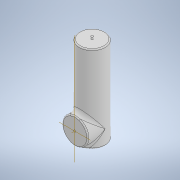
# Autodesk Inventor part: Link3
Saved by Autodesk Inventor 2021 (Build 250183000, 183)
## iProperties
Created: 2021-03-25
Part Number: Link3
Material: 일반
Document SubType Name: Modeling
Designer: jglee
Density: 1 g/cm^3
Appearance: 기본값
Author: jglee
Autodesk Inventor part; units mm, degrees
ref_plane "YZ Plane" through (0, 0, 0) normal (1, 0, 0) x (0, 1, 0)
ref_plane "XZ Plane" through (0, 0, 0) normal (0, 1, 0) x (-1, 0, 0)
ref_plane "XY Plane" through (0, 0, 0) normal (0, 0, 1) x (1, 0, 0)
sketch "스케치1" plane through (0, 0, 0) normal (0, 0, 1) x (1, 0, 0)
  circle A0 centre (0, 0) radius 60
  dimension "d0" = 120
  constraints: 1 centre point, 1 coincident
  measures "d0" diameter of A0
extrude "돌출1" add sketch "스케치1" against normal blind 80
sketch "스케치2" plane through (0, 0, 0) normal (0, 1, 0) x (-1, 0, 0)
  line L0 (-60, -80) -> (60, -80) projected
  circle A0 centre (0, -80) radius 60
  point P0 (0, 0)
  dimension "d3" = 120
  constraints: 1 centre point, 1 midpoint
  measures "d3" diameter of A0
extrude "돌출2" add sketch "스케치2" along normal blind 330 and the other way blind 70
sketch "스케치3" plane through (0, 0, 0) normal (0, 0, 1) x (1, 0, 0)
  circle A0 centre (0, 0) radius 5
  dimension "d8" = 10
  constraints: 1 centre point, 1 coincident
  measures "d8" diameter of A0
extrude "돌출3" cut sketch "스케치3" against normal blind 10
sketch "스케치4" plane through (0, 330, -80) normal (0, 1, 0) x (1, 0, 0)
  circle A0 centre (0, 0) radius 5
  point P0 (0, -80)
  dimension "d11" = 10
  constraints: 1 centre point
  measures "d11" diameter of A0
extrude "돌출4" add sketch "스케치4" along normal blind 10
fillet "모깎기1" radius 20 4 edges at (42.4264, -42.4264, -37.5736) (-42.4264, -42.4264, -37.5736) (-42.4264, 42.4264, -37.5736) (42.4264, 42.4264, -37.5736)
fillet "모깎기2" radius 5 7 edges at (60, 0, 0) (-60, 0, 0) (-14.5209, -70, -20.3078) (14.5231, -70, -20.3086) (30.4726, -70, -131.6858) (-51.6858, -70, -49.5274) (60, 330, -80)
